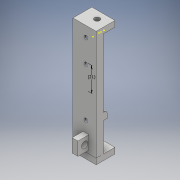
# Autodesk Inventor part: mtv_axelHolder(brakingAxel)2-6
Saved by Autodesk Inventor 2018 (Build 220112000, 112)
## iProperties
Created: 2019-01-14
Part Number: mtv_axelHolder(brakingAxel)2-6
Material: Generic
Document SubType Name: Modeling
Designer: aditya
Density: 1 g/cm^3
Appearance: Default
Author: aditya
## iProperties of the stored document mtv_axelHolder(brakingAxel)1-13_3DPrint.ipt
Created: 2019-01-14
Part Number: mtv_axelHolder(brakingAxel)1-13_3DPrint
Material: Generic
Document SubType Name: Modeling
Designer: aditya
Density: 1 g/cm^3
Appearance: Default
Author: aditya
Autodesk Inventor part; units mm, degrees
ref_plane "YZ Plane" through (0, 0, 0) normal (1, 0, 0) x (0, 1, 0)
ref_plane "XZ Plane" through (0, 0, 0) normal (0, 1, 0) x (-1, 0, 0)
ref_plane "XY Plane" through (0, 0, 0) normal (0, 0, 1) x (1, 0, 0)
sketch "Sketch1" plane through (0, 0, 0) normal (0, 1, 0) x (-1, 0, 0)
  line L0 (0, 0) -> (22.65, 0)
  line L1 (22.65, 0) -> (22.65, -100)
  line L2 (22.65, -100) -> (0, -100)
  line L3 (0, -100) -> (0, 0)
  dimension "d0" = 22.65
  dimension "d1" = 100
  constraints: 8 end point, 2 parallel, 1 horizontal, 1 perpendicular
  measures "d0" distance of L1.end L2.end
  measures "d1" distance of L0.end L1.end
extrude "Extrusion1" add sketch "Sketch1" along normal blind 5
sketch "Sketch2" plane through (0, 5, 0) normal (0, 1, 0) x (1, 0, 0)
  line L0 (-22.65, 0) -> (0, 0) projected
  line L1 (0, 0) -> (0, 100) projected
  line L2 (-22.65, 0) -> (0, 0)
  line L3 (0, 0) -> (0, 5)
  line L4 (0, 5) -> (-22.65, 5)
  line L5 (-22.65, 5) -> (-22.65, 0)
  line L6 (-22.65, 100) -> (-22.65, 0) projected
  line L7 (-22.65, 100) -> (0, 100)
  line L8 (0, 100) -> (0, 95)
  line L9 (0, 95) -> (-22.65, 95)
  line L10 (-22.65, 95) -> (-22.65, 100)
  dimension "d4" = 5
  dimension "d5" = 5
  constraints: 16 end point, 4 parallel, 2 horizontal, 2 perpendicular, 2 point on line
  measures "d4" distance of L3.end L2.end
  measures "d5" distance of L7.end L8.end
extrude "Extrusion2" add sketch "Sketch2" along normal blind 40 contours L5 L4 L1 L0 | L6 L7 L1 L9
sketch "Sketch3" plane through (-22.65, 0, 0) normal (0, 0, 1) x (1, 0, 0)
  point P0 (22.65, 0)
sketch "Sketch4" plane through (-22.65, 0, 0) normal (0, 0, 1) x (1, 0, 0)
  line L0 (22.65, 0) -> (0, 0) projected
  line L1 (22.65, 0) -> (0, 0)
  line L2 (0, 0) -> (11.325, 0)
  line L3 (11.325, 0) -> (11.325, 45)
  line L4 (22.65, 45) -> (0, 45) projected
  line L5 (0, 5) -> (22.65, 5) projected
  line L6 (22.65, 5) -> (0, 5)
  line L7 (11.325, 5) -> (11.325, 15) construction
  dimension "d8" = 10
  constraints: 10 end point, 3 midpoint, 1 collinear, 1 horizontal, 1 point on line
  measures "d8" distance of L7.start L7.end
hole "Hole1" at (-11.325, 15, 0) direction (0, 0, -1) diameter 4 depth 115 tip angle 118
sketch "Sketch5" plane through (-22.65, 0, 0) normal (0, 0, 1) x (1, 0, 0)
  line L0 (0, 5) -> (0, 45)
  line L1 (0, 45) -> (23, 45)
  line L2 (23, 45) -> (23, 21.753841)
  line L3 (23, 21.753841) -> (0, 21.753841)
  line L4 (0, 21.753841) -> (0, 45)
  point P0 (22.65, 0)
  dimension "d16" = 23
  constraints: 8 end point, 2 parallel, 1 horizontal, 1 perpendicular
  measures "d16" distance of L2.end L3.end
extrude "Extrusion3" cut sketch "Sketch5" against normal blind 102.75
sketch "Sketch6" plane through (0, 5, 0) normal (0, 1, 0) x (1, 0, 0)
  line L0 (0, 95) -> (-22.65, 95) construction
  line L1 (-22.65, 5) -> (0, 5) construction
  line L2 (0, 95) -> (0, 5) construction
  line L3 (0, 5) -> (-1.175, 5) construction
  line L4 (-1.175, 5) -> (-1.175, 95) construction
  line L5 (-1.175, 50) -> (-22.65, 50) construction
  line L6 (-22.65, 95) -> (-22.65, 5) construction
  line L7 (0, 5) -> (0, 95) construction
  line L8 (0, 5) -> (-22.65, 5) construction
  line L9 (-13.325, 5) -> (-9.325, 5) construction
  line L10 (-11.325, 5) -> (-11.325, 95) construction
  line L11 (-11.325, 50) -> (-2.825, 50) construction
  line L12 (-2.825, 50) -> (-2.825, 71) construction
  line L13 (-11.325, 50) -> (-19.825, 50) construction
  line L14 (-11.325, 50) -> (-2.825, 50) construction
  line L15 (-19.825, 50) -> (-19.825, 29) construction
  point P0 (0, 0)
  dimension "d19" = 1.175
  dimension "d20" = 8.5
  dimension "d21" = 21
  dimension "d22" = 90
  dimension "d23" = 8.5
  dimension "d24" = 180
  dimension "d25" = 21
  constraints: 22 end point, 5 midpoint, 3 coincident, 2 collinear, 2 parallel, 2 perpendicular, 2 point on line, 1 horizontal, 1 vertical
  measures "d19" distance of L1.end L3.end
  measures "d20" distance of L11.start L11.end
  measures "d21" distance of L11.end L12.end
  measures "d22" angle of L12 L11
  measures "d23" distance of L11.start L13.end
  measures "d24" angle of L13 L14
  measures "d25" distance of L13.end L15.end
hole "Hole2" at (-2.825, 5, -71) at (-19.825, 5, -29) direction (0, -1, 0) diameter 4 depth 115 tip angle 118
fillet "Fillet1" radius 1 2 edges at (-2.825, 5, -73) (-19.825, 5, -31)
sketch "Sketch7" plane through (0, 5, 0) normal (0, 1, 0) x (1, 0, 0)
  circle A0 centre (-2.825, 71) radius 2 construction
  line L0 (-2.825, 71) -> (-22.65, 71) construction
  line L1 (-22.65, 0) -> (-22.65, 100) construction
  circle A1 centre (-19.825, 29) radius 2 construction
  line L2 (-19.825, 29) -> (-19.825, 32.5) construction
  line L3 (-19.825, 32.5) -> (-35.65, 32.5) construction
  line L4 (-22.65, 32.5) -> (-32.65, 32.5) construction
  line L5 (-32.65, 32.5) -> (-32.65, 42.5) construction
  line L6 (-32.65, 42.5) -> (-22.65, 42.5) construction
  line L7 (-22.65, 42.5) -> (-22.65, 32.5) construction
  line L8 (-22.65, 42.5) -> (-32.65, 42.5)
  line L9 (-32.65, 42.5) -> (-32.65, 32.5)
  line L10 (-32.65, 32.5) -> (-22.65, 32.5)
  line L11 (-22.65, 32.5) -> (-22.65, 42.5)
  point P0 (0, 0)
  dimension "d34" = 3.5
  dimension "d35" = 15.825
  dimension "d36" = 10
  dimension "d37" = 10
  constraints: 22 end point, 4 horizontal, 4 parallel, 3 point on line, 2 perpendicular, 1 vertical
  measures "d34" distance of L2.start L2.end
  measures "d35" distance of L2.end L3.end
  measures "d36" distance of L5.end L6.end
  measures "d37" distance of L4.end L5.end
extrude "Extrusion4" add sketch "Sketch7" against normal blind 5
sketch "Sketch8" plane through (0, 5, 0) normal (0, 1, 0) x (1, 0, 0)
  line L0 (-32.65, 42.5) -> (-22.65, 42.5) projected
  line L1 (-22.65, 32.5) -> (-32.65, 32.5) projected
  line L2 (-32.65, 42.5) -> (-27.65, 42.5)
  line L3 (-27.65, 42.5) -> (-27.65, 32.5)
  line L4 (-27.65, 32.5) -> (-32.65, 32.5)
  line L5 (-32.65, 32.5) -> (-32.65, 42.5)
  point P0 (0, 0)
  dimension "d40" = 5
  constraints: 8 end point, 2 parallel, 1 horizontal, 1 midpoint, 1 perpendicular
  measures "d40" distance of L3.end L4.end
extrude "Extrusion5" add sketch "Sketch8" along normal blind 12.5
sketch "Sketch9" plane through (-32.65, 0, -42.5) normal (-1, 0, 0) x (0, 0, 1)
  line L0 (0, 17.5) -> (0, 0) construction
  line L1 (0, 17.5) -> (5, 17.5) construction
  line L2 (10, 17.5) -> (0, 17.5) construction
  line L3 (10, 0) -> (0, 0) construction
  line L4 (5, 0) -> (5, 17.5) construction
  point P0 (42.5, 0)
  point P1 (5, 12.5)
  constraints: 4 end point, 2 midpoint, 1 perpendicular, 1 point on line
hole "Hole3" at (-32.65, 12.5, -37.5) direction (1, 0, 0) diameter 6 depth 115 tip angle 118
fillet "Fillet2" radius 0.1 4 edges at (-22.65, 21.7538, -97.5) (-22.65, 21.7538, -2.5) (0, 21.7538, -2.5) (0, 21.7538, -97.5)
sketch "Sketch10" plane through (-22.65, 0, 0) normal (0, 0, 1) x (1, 0, 0)
  circle A0 centre (11.325, 15) radius 2 projected
  circle A1 centre (11.325, 15) radius 2.125
  point P0 (22.65, 0)
  dimension "d51" = 4.25
  constraints: 1 centre point, 1 coincident
  measures "d51" diameter of A1
extrude "Extrusion6" cut sketch "Sketch10" against normal blind 1000 contours A0 | A1
sketch "Sketch11" plane through (-22.65, 5, -95) normal (0, 0, 1) x (1, 0, 0)
  circle A0 centre (11.325, 10) radius 2.125 construction
  line L0 (11.325, 10) -> (11.325, 6.7) construction
  line L1 (11.325, 6.7) -> (16.825, 6.7) construction
  line L2 (16.825, 6.7) -> (20.025, 6.7) construction
  line L3 (20.025, 6.7) -> (20.025, 3.7) construction
  line L4 (20.025, 3.7) -> (16.825, 3.7) construction
  line L5 (16.825, 3.7) -> (16.825, 6.7) construction
  line L6 (16.825, 6.7) -> (20.025, 6.7)
  line L7 (20.025, 6.7) -> (20.025, 4.6)
  line L8 (20.025, 4.6) -> (16.825, 4.6)
  line L9 (16.825, 4.6) -> (16.825, 6.7)
  point P0 (22.65, -5)
  dimension "d54" = 3.3
  dimension "d55" = 5.5
  dimension "d56" = 3.2
  dimension "d57" = 3
  dimension "d58" = 2.1
  constraints: 20 end point, 4 parallel, 3 perpendicular, 2 horizontal, 1 point on line, 1 vertical
  measures "d54" distance of L0.start L0.end
  measures "d55" distance of L0.end L1.end
  measures "d56" distance of L3.end L4.end
  measures "d57" distance of L2.end L3.end
  measures "d58" distance of L6.end L7.end
extrude "Extrusion7" add sketch "Sketch11" along normal blind 91.25
sketch "Sketch12" plane through (-22.65, 5, -95) normal (0, 0, 1) x (1, 0, 0)
  circle A0 centre (11.325, 10) radius 2.125 construction
  line L0 (11.325, 10) -> (11.325, 5.56) construction
  line L1 (11.325, 5.56) -> (6.325, 5.56) construction
  line L2 (6.325, 5.56) -> (3.574879, 5.56)
  line L3 (3.574879, 5.56) -> (3.574879, 4.56)
  line L4 (3.574879, 4.56) -> (6.325, 4.56)
  line L5 (6.325, 4.56) -> (6.325, 5.56)
  point P0 (22.65, -5)
  dimension "d61" = 4.44
  dimension "d62" = 5
  dimension "d63" = 1
  constraints: 12 end point, 2 parallel, 2 perpendicular, 1 horizontal, 1 vertical
  measures "d61" distance of L0.start L0.end
  measures "d62" distance of L0.end L1.end
  measures "d63" distance of L3.end L2.end
extrude "Extrusion8" add sketch "Sketch12" along normal blind 91.25
sketch "Sketch13" plane through (-5.825, 11.7, -95) normal (0, 1, 0) x (1, 0, 0)
  line L0 (3.2, 0) -> (3.2, -90) projected
  line L1 (0, -25) -> (3.2, -25)
  line L2 (3.2, -25) -> (3.2, -31.35)
  line L3 (3.2, -31.35) -> (0, -31.35)
  line L4 (0, -31.35) -> (0, -25)
  point P0 (5.825, -95)
  dimension "d66" = 6.35
  constraints: 8 end point, 2 parallel, 1 horizontal, 1 perpendicular, 1 point on line
  measures "d66" distance of L1.end L2.end
extrude "Extrusion9" add sketch "Sketch13" along normal blind 3.8
sketch "Sketch14" plane through (0, 5, 0) normal (0, 1, 0) x (1, 0, 0)
  circle A0 centre (-19.825, 29) radius 2 construction
  line L0 (0, 100) -> (0, 0) construction
  circle A1 centre (-2.825, 71) radius 2 construction
  line L1 (-2.825, 71) -> (-22.65, 71) construction
  line L2 (-22.65, 95) -> (-22.65, 42.5) construction
  line L3 (0, 71) -> (-22.65, 71) construction
  line L4 (0, 29) -> (-22.65, 29) construction
  line L5 (-22.65, 29) -> (-11.325, 29) construction
  line L6 (-11.325, 71) -> (-11.325, 29) construction
  constraints: 10 end point, 3 point on line, 2 coincident, 2 midpoint, 2 perpendicular, 1 horizontal
hole "Hole4" at (-11.325, 5, -29) at (-11.325, 5, -71) direction (0, -1, 0) diameter 3.3 depth 8 tip angle 118
sketch "Sketch15" plane through (0, 5, 0) normal (0, 1, 0) x (1, 0, 0)
  line L0 (0, 5) -> (0, 69.990359)
  line L1 (-22.65, 42.5) -> (-22.65, 100)
  line L2 (0, 5) -> (-22.65, 5)
  line L3 (-22.65, 5) -> (-22.65, 94.999965)
  line L4 (-22.65, 94.999965) -> (0, 94.999965)
  line L5 (0, 94.999965) -> (0, 5)
  point P0 (0, 0)
  constraints: 8 end point, 2 parallel, 1 horizontal, 1 perpendicular, 1 point on line
extrude "Extrusion10" add sketch "Sketch15" along normal blind 4.55
sketch "Sketch16" plane through (0, 0, 0) normal (0, -1, 0) x (1, 0, 0)
  circle A0 centre (-11.325, -71) radius 1.65 projected
  circle A1 centre (-11.325, -71) radius 1.65
  circle A2 centre (-11.325, -29) radius 1.65 projected
  circle A3 centre (-11.325, -29) radius 1.65
  point P0 (0, 0)
  constraints: 2 centre point, 2 coincident
hole "Hole5" at (-11.325, 0, -71) at (-11.325, 0, -29) direction (0, 1, 0) diameter 3.3 depth 80 tip angle 118
sketch "Sketch17" plane through (0, 0, -100) normal (0, 0, -1) x (-1, 0, 0)
  line L0 (22.65, 0) -> (0, 0)
  line L1 (22.65, 0) -> (22.65, 21.653841)
  line L2 (0, 0) -> (22.65, 0)
  line L3 (22.65, 0) -> (22.65, 5.45)
  line L4 (22.65, 5.45) -> (0, 5.45)
  line L5 (0, 5.45) -> (0, 0)
  dimension "d85" = 5.45
  constraints: 8 end point, 2 parallel, 1 horizontal, 1 perpendicular, 1 point on line
  measures "d85" distance of L3.end L2.end
extrude "Extrusion11" cut sketch "Sketch17" against normal blind 129.8
sketch "Sketch18" plane through (0, 9.55, 0) normal (0, 1, 0) x (1, 0, 0)
  line L0 (-19.075121, 95) -> (-16.325, 95)
  line L1 (0, 5) -> (-22.65, 5)
  line L2 (-16.325, 95) -> (-5.825, 95)
  line L3 (-5.825, 95) -> (-5.825, 5)
  line L4 (-5.825, 5) -> (-16.325, 5)
  line L5 (-16.325, 5) -> (-16.325, 95)
  point P0 (0, 0)
  dimension "d88" = 10.5
  constraints: 8 end point, 2 parallel, 1 horizontal, 1 perpendicular, 1 point on line
  measures "d88" distance of L3.end L4.end
extrude "Extrusion12" cut sketch "Sketch18" against normal blind 2.5
sketch "Sketch19" plane through (0, 5, 0) normal (0, 1, 0) x (1, 0, 0)
  line L0 (-27.65, 42.5) -> (-27.65, 32.5)
  line L1 (-22.65, 94.999965) -> (-22.65, 5)
  line L2 (-27.65, 42.5) -> (-22.65, 42.5)
  line L3 (-22.65, 42.5) -> (-22.65, 32.5)
  line L4 (-22.65, 32.5) -> (-27.65, 32.5)
  line L5 (-27.65, 32.5) -> (-27.65, 42.5)
  point P0 (0, 0)
  dimension "d91" = 10
  constraints: 8 end point, 2 parallel, 1 horizontal, 1 perpendicular, 1 point on line
  measures "d91" distance of L2.end L3.end
extrude "Extrusion13" add sketch "Sketch19" along normal blind 4.5
sketch "Sketch20" plane through (0, 17.5, 0) normal (0, 1, 0) x (1, 0, 0)
  line L0 (-32.65, 42.5) -> (-32.65, 32.5) projected
  line L1 (-22.65, 42.5) -> (-22.65, 32.5) projected
  line L2 (-32.65, 42.5) -> (-22.65, 42.5)
  line L3 (-22.65, 42.5) -> (-22.65, 32.5)
  line L4 (-22.65, 32.5) -> (-32.65, 32.5)
  line L5 (-32.65, 32.5) -> (-32.65, 42.5)
  point P0 (0, 0)
  constraints: 8 end point, 2 parallel, 1 horizontal, 1 perpendicular
extrude "Extrusion14" cut sketch "Sketch20" against normal blind 8
sketch "Sketch21" plane through (0, 9.55, 0) normal (0, 1, 0) x (1, 0, 0)
  line L0 (-22.65, 32.5) -> (-22.65, 0) construction
  line L1 (-19.075121, 95) -> (-19.075121, 5) construction
  line L2 (-22.65, 32.5) -> (-19.075121, 32.5) construction
  line L3 (-19.075121, 32.5) -> (-19.075121, 42.466168) construction
  line L4 (-19.075121, 42.466168) -> (-22.65, 42.466168) construction
  line L5 (-22.65, 42.466168) -> (-22.65, 32.5) construction
  point P0 (0, 0)
  constraints: 8 end point, 2 parallel, 1 horizontal, 1 perpendicular, 1 point on line
sketch "Sketch22" plane through (0, 9.5, 0) normal (0, 1, 0) x (1, 0, 0)
  line L0 (-32.65, 42.5) -> (-22.65, 42.5) projected
  line L1 (-22.65, 32.5) -> (-22.65, 0) projected
  line L2 (-32.65, 42.5) -> (-22.65, 42.5)
  line L3 (-22.65, 42.5) -> (-22.65, 32.5)
  line L4 (-22.65, 32.5) -> (-32.65, 32.5)
  line L5 (-32.65, 32.5) -> (-32.65, 42.5)
  point P0 (0, 0)
  constraints: 8 end point, 2 parallel, 1 horizontal, 1 perpendicular
extrude "Extrusion15" cut sketch "Sketch22" against normal blind 15.5
sketch "Sketch23" plane through (0, 9.55, 0) normal (0, 1, 0) x (1, 0, 0)
  point P0 (0, 0)
sketch "Sketch24" plane through (0, 9.55, 0) normal (0, 1, 0) x (1, 0, 0)
  line L0 (-22.65, 94.999965) -> (-22.65, 0)
  line L1 (-22.65, 32.500017) -> (-32.65, 32.500017)
  line L2 (-32.65, 32.500017) -> (-32.65, 42.500017)
  line L3 (-32.65, 42.500017) -> (-22.65, 42.500017)
  line L4 (-22.65, 42.500017) -> (-22.65, 32.500017)
  point P0 (0, 0)
  dimension "d98" = 10
  dimension "d99" = 10
  constraints: 8 end point, 2 parallel, 1 horizontal, 1 perpendicular, 1 point on line
  measures "d98" distance of L2.end L3.end
  measures "d99" distance of L1.end L2.end
extrude "Extrusion16" add sketch "Sketch24" against normal blind 4.1
sketch "Sketch25" plane through (-32.65, 9.55, -32.500017) normal (0, 0, 1) x (1, 0, 0)
  line L0 (0, 0) -> (0, -4.1) projected
  line L1 (0, -4.1) -> (5, -4.1)
  line L2 (5, -4.1) -> (5, 13.4)
  line L3 (5, 13.4) -> (0, 13.4)
  line L4 (0, 13.4) -> (0, -4.1)
  point P0 (32.65, -9.55)
  dimension "d102" = 5
  dimension "d103" = 17.5
  constraints: 8 end point, 2 parallel, 1 horizontal, 1 perpendicular
  measures "d102" distance of L3.end L2.end
  measures "d103" distance of L2.end L1.end
extrude "Extrusion17" add sketch "Sketch25" against normal blind 10
sketch "Sketch26" plane through (-32.65, 5.45, -42.500017) normal (-1, 0, 0) x (0, 0, 1)
  line L0 (10, 17.5) -> (0, 17.5) construction
  line L1 (0, 17.5) -> (10, 17.5) construction
  line L2 (10, 17.5) -> (5, 17.5) construction
  line L3 (5, 17.5) -> (5, 12.5) construction
  point P0 (42.500017, -5.45)
  dimension "d106" = 5
  constraints: 6 end point, 1 collinear, 1 midpoint, 1 perpendicular
  measures "d106" distance of L2.end L3.end
hole "Hole6" at (-32.65, 17.95, -37.500017) direction (1, 0, 0) diameter 6 depth 80 tip angle 118
fillet "Fillet3" radius 2 2 edges at (-11.325, 7.05, -27.35) (-11.325, 7.05, -69.35)
sketch "Sketch27" plane through (0, 9.55, 0) normal (0, 1, 0) x (1, 0, 0)
  line L0 (0, 5) -> (0, 94.999965)
  line L1 (-2.625, 95) -> (-2.625, 5)
  line L2 (0, 94.999965) -> (-2.625, 94.999965)
  line L3 (-2.625, 94.999965) -> (-2.625, 5)
  line L4 (-2.625, 5) -> (0, 5)
  line L5 (0, 5) -> (0, 94.999965)
  line L6 (-22.55, 100) -> (-0.1, 100)
  line L7 (0, 0) -> (-2.625, 0)
  line L8 (-2.625, 0) -> (-2.625, 100)
  line L9 (-2.625, 100) -> (0, 100)
  line L10 (0, 100) -> (0, 0)
  constraints: 16 end point, 4 parallel, 2 horizontal, 2 perpendicular, 1 point on line
extrude "Extrusion18" cut sketch "Sketch27" along normal mid plane 45
sketch "Sketch28" plane through (0, 7.05, 0) normal (0, 1, 0) x (1, 0, 0)
  circle A0 centre (-11.325, 71) radius 1.65 construction
  circle A1 centre (-11.325, 29) radius 1.65 construction
  line L0 (-11.325, 71) -> (-11.325, 29) construction
  line L1 (-11.325, 29) -> (-11.325, 50) construction
  line L2 (-11.325, 50) -> (-22.65, 50) construction
  line L3 (-22.65, 94.999965) -> (-22.65, 42.500017) construction
  point P0 (0, 0)
  dimension "d117" = 21
  constraints: 6 end point, 1 midpoint, 1 perpendicular, 1 point on line, 1 vertical
  measures "d117" distance of L0.end L1.end
sketch "Sketch29" plane through (-2.625, 21.753841, -100) normal (0, 0, -1) x (-1, 0, 0)
  circle A0 centre (8.7, -6.753841) radius 2.125
  circle A1 centre (8.7, -6.753841) radius 2.25
  point P0 (-2.625, -21.753841)
  dimension "d118" = 4.5
  constraints: 1 centre point, 1 coincident
  measures "d118" diameter of A1
extrude "Extrusion19" cut sketch "Sketch29" against normal blind 118 contours A0 | A1
sketch "Sketch30" plane through (0, 9.55, 0) normal (0, 1, 0) x (1, 0, 0)
  line L0 (-2.625, 100) -> (-22.65, 100) construction
  line L1 (-22.65, 0) -> (-2.625, 0) construction
  line L2 (-2.625, 100) -> (-2.625, 0) construction
  line L3 (-2.625, 0) -> (-2.625, 50) construction
  line L4 (-2.625, 50) -> (-22.65, 50) construction
  line L5 (-22.65, 94.999965) -> (-22.65, 42.500017) construction
  line L6 (-22.65, 50) -> (-22.65, 57.5) construction
  line L7 (-22.65, 57.5) -> (-32.65, 57.5)
  line L8 (-32.65, 57.5) -> (-32.65, 67.5)
  line L9 (-32.65, 67.5) -> (-22.65, 67.5)
  line L10 (-22.65, 67.5) -> (-22.65, 57.5)
  point P0 (0, 0)
  dimension "d121" = 50
  dimension "d122" = 7.49998
  dimension "d123" = 7.5
  dimension "d124" = 10
  dimension "d125" = 10
  constraints: 16 end point, 3 perpendicular, 2 parallel, 2 point on line, 1 horizontal, 1 midpoint
  measures "d121" distance of L1.end L3.end
  measures "d122" distance of L5.end L4.end
  measures "d123" distance of L4.end L6.end
  measures "d124" distance of L8.end L9.end
  measures "d125" distance of L7.end L8.end
extrude "Extrusion20" add sketch "Sketch30" against normal blind 4.1
sketch "Sketch31" plane through (0, 9.55, 0) normal (0, 1, 0) x (1, 0, 0)
  line L0 (-32.65, 57.5) -> (-32.65, 67.5) projected
  line L1 (-22.65, 57.5) -> (-32.65, 57.5) projected
  line L2 (-32.65, 67.5) -> (-27.65, 67.5)
  line L3 (-27.65, 67.5) -> (-27.65, 57.5)
  line L4 (-27.65, 57.5) -> (-32.65, 57.5)
  line L5 (-32.65, 57.5) -> (-32.65, 67.5)
  point P0 (0, 0)
  constraints: 8 end point, 2 parallel, 1 horizontal, 1 midpoint, 1 perpendicular
extrude "Extrusion21" add sketch "Sketch31" along normal blind 13.4
sketch "Sketch32" plane through (-32.65, 5.45, -67.5) normal (-1, 0, 0) x (0, 0, 1)
  line L0 (0, 17.5) -> (10, 17.5) construction
  line L1 (5, 17.5) -> (5, 12.5) construction
  point P0 (67.5, -5.45)
  dimension "d130" = 5
  constraints: 2 end point, 1 midpoint, 1 vertical
  measures "d130" distance of L1.start L1.end
hole "Hole7" at (-32.65, 17.95, -62.5) direction (1, 0, 0) diameter 6 depth 8 tip angle 118
sketch "Sketch33" plane through (-32.65, 22.95, -32.500017) normal (0, 1, 0) x (1, 0, 0)
  line L0 (10, 24.999983) -> (10, 10)
  line L1 (0, 0) -> (0, 10)
  line L2 (10, 10) -> (0, 10)
  line L3 (0, 10) -> (0, 0)
  line L4 (0, 0) -> (10, 0)
  line L5 (10, 0) -> (10, 10)
  point P0 (32.65, -32.500017)
  constraints: 8 end point, 2 parallel, 1 horizontal, 1 perpendicular
extrude "Extrusion22" cut sketch "Sketch33" against normal blind 130.4
sketch "Sketch34" plane through (-2.625, 11.7, -95) normal (1, 0, 0) x (0, 0, -1)
  line L0 (-31.35, 0) -> (-31.35, 3.8) projected
  line L1 (-31.35, 3.8) -> (-31.35, 2.8)
  line L2 (-25, 0) -> (-25, 3.8) construction
  line L3 (-25, 3.8) -> (-26, 3.8) construction
  line L4 (-31.35, 3.8) -> (-25, 3.8) construction
  line L5 (-31.35, 2.8) -> (-26, 3.8)
  line L6 (-31.35, 3.8) -> (-26, 3.8)
  point P0 (-95, -11.7)
  dimension "d140" = 1
  dimension "d141" = 1
  constraints: 8 end point, 2 point on line, 1 collinear
  measures "d140" distance of L0.end L1.end
  measures "d141" distance of L2.end L3.end
extrude "Extrusion23" cut sketch "Sketch34" against normal blind 3.85
fillet "Fillet4" radius 3 1 edges at (-4.225, 15.5, -69)
fillet "Fillet5" radius 2 1 edges at (-4.225, 14.5, -63.65)
sketch "Sketch35" plane through (0, 22.95, 0) normal (0, 1, 0) x (1, 0, 0)
  line L0 (-22.65, 57.5) -> (-32.65, 57.5)
  line L1 (-22.65, 94.999965) -> (-22.65, 67.5)
  line L2 (-32.65, 57.5) -> (-22.65, 57.5)
  line L3 (-22.65, 57.5) -> (-22.65, 67.5)
  line L4 (-22.65, 67.5) -> (-32.65, 67.5)
  line L5 (-32.65, 67.5) -> (-32.65, 57.5)
  point P0 (0, 0)
  constraints: 8 end point, 2 parallel, 1 horizontal, 1 perpendicular
extrude "Extrusion24" cut sketch "Sketch35" against normal blind 100
sketch "Sketch36" plane through (-22.65, 5.45, -94.999965) normal (0, -1, 0) x (1, 0, 0)
  circle A0 centre (11.325, 23.999965) radius 1.65 construction
  line L0 (11.325, 23.999965) -> (11.325, 19.999965) construction
  line L1 (11.325, 19.999965) -> (20.025, 19.999965) construction
  line L2 (20.025, -0.000035) -> (20.025, 24.999965) construction
  line L3 (0, 0) -> (0, 89.999965) construction
  line L4 (0, 19.999965) -> (20.025, 19.999965) construction
  line L5 (11.325, 19.999965) -> (11.325, 9.999965) construction
  line L6 (13.825, 19.999965) -> (8.825, 9.999965) construction
  line L7 (8.825, 19.999965) -> (13.825, 9.999965) construction
  line L8 (8.825, 19.999965) -> (13.825, 19.999965) construction
  line L9 (13.825, 19.999965) -> (13.825, 4.999965) construction
  line L10 (13.825, 4.999965) -> (8.825, 4.999965) construction
  line L11 (8.825, 4.999965) -> (8.825, 19.999965) construction
  line L12 (8.825, 4.999965) -> (13.825, 4.999965)
  line L13 (13.825, 4.999965) -> (13.825, 12.499965)
  line L14 (13.825, 12.499965) -> (8.825, 12.499965)
  line L15 (8.825, 12.499965) -> (8.825, 4.999965)
  point P0 (22.65, 94.999965)
  point P1 (11.325, 14.999965)
  dimension "d148" = 4
  dimension "d149" = 10
  dimension "d150" = 5
  dimension "d151" = 15
  dimension "d152" = 7.5
  constraints: 28 end point, 4 midpoint, 4 parallel, 3 perpendicular, 3 point on line, 2 horizontal, 2 vertical, 1 collinear
  measures "d148" distance of L0.start L0.end
  measures "d149" distance of L0.end L5.end
  measures "d150" distance of L7.end L6.end
  measures "d151" distance of L8.end L9.end
  measures "d152" distance of L13.end L12.end
extrude "Extrusion25" add sketch "Sketch36" along normal blind 7.5
sketch "Sketch37" plane through (-13.825, 5.45, -90) normal (-1, 0, 0) x (0, 0, 1)
  line L0 (0, 0) -> (0, -7.5) construction
  line L1 (7.5, 0) -> (0, 0) construction
  line L2 (0, -7.5) -> (7.5, 0) construction
  line L3 (0, -7.5) -> (7.5, -7.5) construction
  line L4 (7.5, 0) -> (7.5, -7.5) construction
  line L5 (7.5, -7.5) -> (0, 0) construction
  point P0 (90, -5.45)
  point P1 (3.75, -3.75)
  constraints: 6 end point, 2 perpendicular, 1 midpoint
hole "Hole8" at (-13.825, 1.7, -86.25) direction (1, 0, 0) diameter 6 depth 8 tip angle 118
sketch "Sketch38" plane through (-13.825, 5.45, -90) normal (-1, 0, 0) x (0, 0, 1)
  circle A0 centre (3.75, -3.75) radius 3 projected
  circle A1 centre (3.75, -3.75) radius 2.75
  point P0 (90, -5.45)
  dimension "d162" = 5.5
  constraints: 1 centre point, 1 coincident
  measures "d162" diameter of A1
extrude "Extrusion26" add sketch "Sketch38" against normal blind 5
sketch "Sketch39" plane through (-22.65, 5.45, -94.999965) normal (0, -1, 0) x (1, 0, 0)
  point P0 (22.65, 94.999965)
sketch "Sketch40" plane through (-5.825, 11.7, -5) normal (0, 1, 0) x (1, 0, 0)
  line L0 (3.2, 89.999965) -> (-16.825, 89.999965)
  line L1 (0, 89.999965) -> (0, 0)
  line L2 (3.2, 89.999965) -> (0, 89.999965)
  line L3 (0, 89.999965) -> (0, 0)
  line L4 (0, 0) -> (3.2, 0)
  line L5 (3.2, 0) -> (3.2, 89.999965)
  point P0 (5.825, -5)
  constraints: 8 end point, 2 parallel, 1 horizontal, 1 perpendicular
extrude "Extrusion27" add sketch "Sketch40" against normal blind 5.5
sketch "Sketch41" plane through (-13.825, 5.45, -82.5) normal (0, 0, 1) x (1, 0, 0)
  line L0 (0, 0) -> (0, -7.5) projected
  line L1 (5, 0) -> (5, -7.5) projected
  line L2 (0, -7.5) -> (5, -7.5)
  line L3 (5, -7.5) -> (5, 0)
  line L4 (5, 0) -> (0, 0)
  line L5 (0, 0) -> (0, -7.5)
  point P0 (13.825, -5.45)
  constraints: 8 end point, 2 parallel, 1 horizontal, 1 perpendicular
extrude "Extrusion28" add sketch "Sketch41" along normal blind 2
sketch "Sketch42" plane through (-8.825, 5.45, -90) normal (0, 0, -1) x (-1, 0, 0)
  line L0 (5, -7.5) -> (0, -7.5) projected
  line L1 (0, -7.5) -> (5, -7.5)
  line L2 (5, -7.5) -> (5, 0)
  line L3 (5, 0) -> (0, 0)
  line L4 (0, 0) -> (0, -7.5)
  point P0 (-8.825, -5.45)
  constraints: 8 end point, 2 parallel, 1 horizontal, 1 perpendicular
extrude "Extrusion29" add sketch "Sketch42" along normal blind 2
sketch "Sketch43" plane through (-22.65, -2.05, -94.999965) normal (0, -1, 0) x (1, 0, 0)
  line L0 (8.825, 14.499965) -> (13.825, 14.499965)
  line L1 (13.825, 14.499965) -> (13.825, 2.999965)
  line L2 (8.825, 14.499965) -> (13.825, 14.499965)
  line L3 (13.825, 14.499965) -> (13.825, 2.999965)
  line L4 (13.825, 2.999965) -> (8.825, 2.999965)
  line L5 (8.825, 2.999965) -> (8.825, 14.499965)
  point P0 (22.65, 94.999965)
  constraints: 8 end point, 2 parallel, 1 horizontal, 1 perpendicular
extrude "Extrusion30" add sketch "Sketch43" along normal blind 2
sketch "Sketch44" plane through (0, 7.05, 0) normal (0, 1, 0) x (1, 0, 0)
  circle A0 centre (-11.325, 29) radius 1.65 construction
  line L0 (-11.325, 29) -> (-11.325, 9) construction
  circle A1 centre (-11.325, 9) radius 1.65
  point P0 (0, 0)
  dimension "d173" = 20
  dimension "d174" = 3.3
  constraints: 2 end point, 1 centre point, 1 coincident, 1 vertical
  measures "d173" distance of L0.start L0.end
  measures "d174" diameter of A1
extrude "Extrusion31" cut sketch "Sketch44" against normal blind 10
fillet "Fillet6" radius 2 1 edges at (-12.975, 7.05, -9)
body "Solid1"
